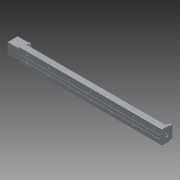
# Autodesk Inventor part: KR55A-980L-1A0-Body
Saved by Autodesk Inventor 2011 SP1 (Build 150282100, 282)
## iProperties
Created: 2013-10-23
Part Number: KR55A-980L-1A0-Body
Catalog Web Link: www.cadenas.de
Description: LM Guide Actuator - Body-KR
Vendor: THK
Document SubType Name: Modeling
Designer: PARTuser1
Manufacturer: THK
Density: 1 g/cm^3
Category: PARTsolutions
Company: THK
Title: KR55A-980L-1A0-Body
Author: Cadenas PARTsolutions
Comments: KR
PSOL_IDENT_0: {$CADENAS_DATA\23d-libs\thk\lm_guide_actuator\type_kr\parts\lm_g_a_kr_body.prj},214 {VTYP=3D},{NB=KR
PSOL_IDENT_1: 55A-980L-1A0-Body},{LINA=KR55A-980L-1A0-Body},{NN=LM Guide Actuator - Body},{DATE=10.01.2013 04:45:2
PSOL_IDENT_2: 4},{GEOMDATE=10.01.2013 04:45:00},{VERSION=},{LINEID=80},{LINESUBID=-1},{WBVAR=LM,TYPE,PC,TOHIF}  {N
PSOL_IDENT_3: B=KR55A-980L-1A0-Body},{LINA=KR55A-980L-1A0-Body},{KT=DUMMY},{ORDER=KR55},{XTYPE=8},{LM=980},{L1=108
PSOL_IDENT_4: 9},{TYPE=A},{SR=826},{H=90},{G=40},{F=200},{N=7},{N1=5},{LM1=980,1080,1180,1280,1380},{TYPE1='A','B'
PSOL_IDENT_5: },{TYPE2=2},{PC=1},{TOHIF=A0},{TOHIF1='A0','Basic Type (with Housing A, without Intermediate flange)
PSOL_IDENT_6: ','00','Old Basic Type (with Housing A, without Intermediate flange)','1[]','Administration number 1
PSOL_IDENT_7: []','0A','Administration number 0A','0B','Administration number 0B','0G','Administration number 0G'}
PSOL_IDENT_8: ,{TOB=1},{DMTR=64},{A=96},{L=976}
CNS_NT: KR
CNS_NB: KR55A-980L-1A0-Body
CNS_NBSYN: $ORDER.$TYPE.-$LM.L-$PC.$TOHIF.-Body
CNS_LINA: KR55A-980L-1A0-Body
CNS_ORDER: KR55
CNS_XTYPE: 8
CNS_LM: 980
CNS_L1: 1089.000
CNS_TYPE: A
CNS_SR: 826.000
CNS_H: 90.000
CNS_G: 40.000
CNS_F: 200.000
CNS_N: 7.000
CNS_N1: 5.000
CNS_LM1: 980,1080,1180,1280,1380
CNS_TYPE1: 'A','B'
CNS_TYPE2: 2.000
CNS_PC: Cover provided
CNS_TOHIF: Basic Type (with Housing A, without Intermediate flange)
CNS_TOHIF1: 'A0','Basic Type (with Housing A, without Intermediate flange)','00','Old Basic Type (with Housing A, without Intermediate flange)','1[]','Administration number 1[]','0A','Administration number 0A','0B','Administration number 0B','0G','Administration number 0G'
CNS_TOB: 1.000
CNS_DMTR: 64.000
CNS_A: 96.000
CNS_L: 976.000
SUPPLIER: THK
ARTICLENO: KR55A-980L-1A0-Body
BOMINFO: KR55A-980L-1A0-Body
CREATOR: CADENAS GmbH
Autodesk Inventor part; units mm, degrees
sketch "Sketch_1" plane through (0, 0, 0) normal (1, 0, 0) x (0, 1, 0)
  line L0 (-30.7, 50) -> (-32, 48.7)
  line L1 (-32, 48.7) -> (-32, 19.7)
  line L2 (-32, 19.7) -> (-31.3, 19)
  line L3 (-31.3, 19) -> (-31.3, 6.3)
  line L4 (-31.3, 6.3) -> (-32, 5.6)
  line L5 (-32, 5.6) -> (-32, -5.6)
  line L6 (-32, -5.6) -> (-31.3, -6.3)
  line L7 (-31.3, -6.3) -> (-31.3, -19)
  line L8 (-31.3, -19) -> (-32, -19.7)
  line L9 (-32, -19.7) -> (-32, -48.7)
  line L10 (-32, -48.7) -> (-30.7, -50)
  line L11 (-30.7, -50) -> (-17.5, -50)
  line L12 (-17.5, -50) -> (-17, -49.5)
  line L13 (-17, -49.5) -> (7, -49.5)
  line L14 (7, -49.5) -> (8, -48.5)
  line L15 (8, -48.5) -> (8, -36.72)
  line L16 (8, -36.72) -> (7.5, -36.22)
  line L17 (7.5, -36.22) -> (3.59, -36.22)
  line L18 (3.59, -36.22) -> (0.49, -39.32)
  line L19 (0.49, -39.32) -> (-11.32, -39.32)
  line L20 (-11.32, -39.32) -> (-14.42, -36.22)
  line L21 (-14.42, -36.22) -> (-15, -36.22)
  arc A0 (-19, -32.22) -> (-15, -36.22) centre (-15, -32.22) ccw
  line L22 (-19, -32.22) -> (-19, 32.22)
  arc A1 (-15, 36.22) -> (-19, 32.22) centre (-15, 32.22) ccw
  line L23 (-15, 36.22) -> (-14.42, 36.22)
  line L24 (-14.42, 36.22) -> (-11.32, 39.32)
  line L25 (-11.32, 39.32) -> (0.49, 39.32)
  line L26 (0.49, 39.32) -> (3.59, 36.22)
  line L27 (3.59, 36.22) -> (7.5, 36.22)
  line L28 (7.5, 36.22) -> (8, 36.72)
  line L29 (8, 36.72) -> (8, 48.5)
  line L30 (8, 48.5) -> (7, 49.5)
  line L31 (7, 49.5) -> (-17, 49.5)
  line L32 (-17, 49.5) -> (-17.5, 50)
  line L33 (-17.5, 50) -> (-30.7, 50)
  constraints: 68 end point, 4 point on circle, 2 centre point
extrude "Extrusion1" add sketch "Sketch_1" along normal blind 980
sketch "Sketch_2" plane through (0, 0, 0) normal (1, 0, 0) x (0, 1, 0)
  line L0 (23, 49.5) -> (-29.5, 49.5)
  arc A0 (-29.5, 49.5) -> (-31.5, 47.5) centre (-29.5, 47.5) ccw
  line L1 (-31.5, 47.5) -> (-31.5, -47.5)
  arc A1 (-31.5, -47.5) -> (-29.5, -49.5) centre (-29.5, -47.5) ccw
  line L2 (-29.5, -49.5) -> (23, -49.5)
  arc A2 (23, -49.5) -> (25, -47.5) centre (23, -47.5) ccw
  line L3 (25, -47.5) -> (25, -43.5)
  arc A3 (25.5, -43) -> (25, -43.5) centre (25.5, -43.5) ccw
  line L4 (25.5, -43) -> (38, -43)
  arc A4 (38, -43) -> (40, -41) centre (38, -41) ccw
  line L5 (40, -41) -> (40, 41)
  arc A5 (40, 41) -> (38, 43) centre (38, 41) ccw
  line L6 (38, 43) -> (25.5, 43)
  arc A6 (25, 43.5) -> (25.5, 43) centre (25.5, 43.5) ccw
  line L7 (25, 43.5) -> (25, 47.5)
  arc A7 (25, 47.5) -> (23, 49.5) centre (23, 47.5) ccw
  constraints: 16 end point, 16 point on circle, 8 centre point
extrude "Extrusion2" add sketch "Sketch_2" against normal blind 15
sketch "Sketch_17" plane through (0, 0, 0) normal (1, 0, 0) x (0, 1, 0)
  line L0 (37, 39) -> (-29.5, 39)
  arc A0 (-29.5, 39) -> (-31.5, 37) centre (-29.5, 37) ccw
  line L1 (-31.5, 37) -> (-31.5, -37)
  arc A1 (-31.5, -37) -> (-29.5, -39) centre (-29.5, -37) ccw
  line L2 (-29.5, -39) -> (37, -39)
  arc A2 (37, -39) -> (40, -36) centre (37, -36) ccw
  line L3 (40, -36) -> (40, 36)
  arc A3 (40, 36) -> (37, 39) centre (37, 36) ccw
  constraints: 8 end point, 8 point on circle, 4 centre point
extrude "Extrusion3" add sketch "Sketch_17" against normal blind 94
sketch "Sketch_3" plane through (0, 0, 0) normal (1, 0, 0) x (0, 1, 0)
  arc A0 (18, 24) -> (-18, 24) centre (0, 0) ccw
  line L0 (-18, 24) -> (-18, -24)
  arc A1 (-18, -24) -> (18, -24) centre (0, 0) ccw
  line L1 (18, -24) -> (18, 24)
  constraints: 4 end point, 4 point on circle, 2 centre point
extrude "Extrusion4" add sketch "Sketch_3" along normal blind 5
sketch "Sketch_4" plane through (0, 0, 0) normal (1, 0, 0) x (0, 1, 0)
  arc A0 (8, 25.7876) -> (-8, 25.7876) centre (0, 0) ccw
  line L0 (-8, 25.7876) -> (-8, 14.8866)
  arc A1 (8, 14.8866) -> (-8, 14.8866) centre (0, 0) ccw
  line L1 (8, 14.8866) -> (8, 25.7876)
  constraints: 4 end point, 4 point on circle, 2 centre point
extrude "Extrusion5" add sketch "Sketch_4" along normal blind 15
sketch "Sketch_26" plane through (0, 0, 0) normal (1, 0, 0) x (0, 1, 0)
  arc A0 (-8, -14.8866) -> (8, -14.8866) centre (0, 0) ccw
  line L0 (-8, -14.8866) -> (-8, -25.7876)
  arc A1 (-8, -25.7876) -> (8, -25.7876) centre (0, 0) ccw
  line L1 (8, -25.7876) -> (8, -14.8866)
  constraints: 4 end point, 4 point on circle, 2 centre point
extrude "Extrusion6" add sketch "Sketch_26" along normal blind 15
sketch "Sketch_38" plane through (0, 12.5, 0) normal (0, 1, 0) x (1, 0, 0)
  line L0 (10, -21.65) -> (5, -21.65)
  line L1 (5, -21.65) -> (5, -17.4)
  line L2 (5, -17.4) -> (9.8, -17.4)
  arc A0 (10, -17.6) -> (9.8, -17.4) centre (9.8, -17.6) ccw
  line L3 (10, -17.6) -> (10, -21.65)
  line L4 (10, -21.65) -> (5, -21.65)
  constraints: 10 end point, 2 point on circle, 1 centre point
revolve "Revolution1" add sketch "Sketch_38" angle 360 about axis through (10, 12.5, 21.65) along (1, 0, 0)
pattern_linear "Rectangular Pattern1" count 2 spacing 43.3 along (0, 0, -1) count 2 spacing 25 along (0, -1, 0) of "Revolution1"
sketch "Sketch_7" plane through (980, 0, 0) normal (1, 0, 0) x (0, 0, -1)
  line L0 (-50, 38.35) -> (-50, -29.85)
  arc A0 (-50, -29.85) -> (-48.35, -31.5) centre (-48.35, -29.85) ccw
  line L1 (-48.35, -31.5) -> (48.35, -31.5)
  arc A1 (48.35, -31.5) -> (50, -29.85) centre (48.35, -29.85) ccw
  line L2 (50, -29.85) -> (50, 38.35)
  arc A2 (50, 38.35) -> (48.35, 40) centre (48.35, 38.35) ccw
  line L3 (48.35, 40) -> (-48.35, 40)
  arc A3 (-48.35, 40) -> (-50, 38.35) centre (-48.35, 38.35) ccw
  constraints: 8 end point, 8 point on circle, 4 centre point
extrude "Extrusion7" add sketch "Sketch_7" along normal blind 15
sketch "Sketch_20" plane through (980, 0, 0) normal (1, 0, 0) x (0, 0, -1)
  line L0 (-55, 18) -> (-43, 18)
  line L1 (-43, 18) -> (-43, 38.35)
  arc A0 (-41.35, 40) -> (-43, 38.35) centre (-41.35, 38.35) ccw
  line L2 (-41.35, 40) -> (41.35, 40)
  arc A1 (43, 38.35) -> (41.35, 40) centre (41.35, 38.35) ccw
  line L3 (43, 38.35) -> (43, 18)
  line L4 (43, 18) -> (55, 18)
  line L5 (55, 18) -> (55, 48)
  line L6 (55, 48) -> (-55, 48)
  line L7 (-55, 48) -> (-55, 18)
  constraints: 16 end point, 4 point on circle, 2 centre point
extrude "Extrusion8" cut sketch "Sketch_20" along normal blind 20
sketch "Sketch_23" plane through (0, 0, 0) normal (0, 0, 1) x (1, 0, 0)
  line L0 (984, 0) -> (979, 0)
  line L1 (979, 0) -> (979, 15)
  line L2 (979, 15) -> (984, 15)
  line L3 (984, 15) -> (984, 0)
  line L4 (984, 0) -> (979, 0)
  constraints: 10 end point
revolve "Revolution2" cut sketch "Sketch_23" angle 360 about axis through (984, 0, 0) along (1, 0, 0)
sketch "Sketch_8" plane through (0, -5, 0) normal (0, 1, 0) x (1, 0, 0)
  line L0 (980, 25) -> (969, 25)
  line L1 (969, 25) -> (969, 32)
  line L2 (969, 32) -> (980, 34)
  line L3 (980, 34) -> (980, 25)
  line L4 (980, 25) -> (969, 25)
  constraints: 10 end point
revolve "Revolution3" add sketch "Sketch_8" angle 360 about axis through (980, -5, -25) along (1, 0, 0)
sketch "Sketch_41" plane through (0, -5, 0) normal (0, 1, 0) x (1, 0, 0)
  line L0 (980, -25) -> (969, -25)
  line L1 (969, -25) -> (969, -18)
  line L2 (969, -18) -> (980, -16)
  line L3 (980, -16) -> (980, -25)
  line L4 (980, -25) -> (969, -25)
  constraints: 10 end point
revolve "Revolution4" add sketch "Sketch_41" angle 360 about axis through (980, -5, 25) along (1, 0, 0)
sketch "Sketch_9" plane through (0, 0, 0) normal (0, 0, 1) x (1, 0, 0)
  line L0 (984, 0) -> (4, 0)
  line L1 (4, 0) -> (4, 10)
  line L2 (4, 10) -> (984, 10)
  line L3 (984, 10) -> (984, 0)
  line L4 (984, 0) -> (4, 0)
  constraints: 10 end point
revolve "Revolution5" add sketch "Sketch_9" angle 360 about axis through (984, 0, 0) along (1, 0, 0)
sketch "Sketch14" plane through (995, 0, 0) normal (1, 0, 0) x (0, 0, -1)
  point P0 (-44.5, -26)
hole "Drilling 2" at (995, -26, 44.5) direction (-1, 0, 0) diameter 7.7 depth 3
pattern_linear "Rectangular Pattern2" count 2 spacing 89 along (0, 0, -1) count 3 spacing 15 along (0, 1, 0) of "Drilling 2"
sketch "Sketch_11" plane through (0, -26, 0) normal (0, 1, 0) x (1, 0, 0)
  line L0 (995, -44.5) -> (991.3, -44.5)
  line L1 (991.3, -44.5) -> (991.3, -41)
  line L2 (991.3, -41) -> (994.8, -41)
  arc A0 (995, -41.2) -> (994.8, -41) centre (994.8, -41.2) ccw
  line L3 (995, -41.2) -> (995, -44.5)
  line L4 (995, -44.5) -> (991.3, -44.5)
  constraints: 10 end point, 2 point on circle, 1 centre point
revolve "Revolution6" add sketch "Sketch_11" angle 360 about axis through (995, -26, 44.5) along (1, 0, 0)
pattern_linear "Rectangular Pattern3" count 2 spacing 89 along (0, 0, -1) count 3 spacing 15 along (0, 1, 0) of "Revolution6"
sketch "Sketch_13" plane through (0, -27, 0) normal (0, 1, 0) x (1, 0, 0)
  arc A0 (-72, -19) -> (-62, -29) centre (-62, -19) ccw
  line L0 (-62, -29) -> (-37, -29)
  arc A1 (-37, -29) -> (-27, -19) centre (-37, -19) ccw
  line L1 (-27, -19) -> (-27, 19)
  arc A2 (-27, 19) -> (-37, 29) centre (-37, 19) ccw
  line L2 (-37, 29) -> (-62, 29)
  arc A3 (-62, 29) -> (-72, 19) centre (-62, 19) ccw
  line L3 (-72, 19) -> (-72, -19)
  constraints: 8 end point, 8 point on circle, 4 centre point
extrude "Extrusion9" cut sketch "Sketch_13" along normal blind 72
sketch "Sketch_39" plane through (0, 0, 0) normal (0, 1, 0) x (-1, 0, 0)
  line L0 (-996, 0) -> (-991, 0)
  line L1 (-994, 0) -> (-994, -7.5)
  line L2 (-994, -7.5) -> (-993, -8.5)
  line L3 (-993, -8.5) -> (-991, -8.5)
  line L4 (-991, -8.5) -> (-991, -15)
  line L5 (-991, -15) -> (-996, -15)
  line L6 (-996, -15) -> (-996, 0)
  line L7 (-996, 0) -> (-994, 0)
  constraints: 16 end point
revolve "Revolution7" cut sketch "Sketch_39" angle 360 about axis through (996, 0, 0) along (1, 0, 0)
sketch "Sketch_18" plane through (0, 0, 0) normal (0, 0, 1) x (1, 0, 0)
  line L0 (-65, 0) -> (-95, 0)
  line L1 (-95, 0) -> (-95, 25)
  line L2 (-95, 25) -> (-65, 25)
  line L3 (-65, 25) -> (-65, 0)
  line L4 (-65, 0) -> (-95, 0)
  constraints: 10 end point
revolve "Revolution8" cut sketch "Sketch_18" angle 360 about axis through (-65, 0, 0) along (1, 0, 0)
sketch "Sketch_19" plane through (0, -26, 0) normal (0, 1, 0) x (1, 0, 0)
  line L0 (-15, -44.5) -> (-20, -44.5)
  line L1 (-20, -44.5) -> (-20, -40.45)
  arc A0 (-19.8, -40.25) -> (-20, -40.45) centre (-19.8, -40.45) ccw
  line L2 (-19.8, -40.25) -> (-15, -40.25)
  line L3 (-15, -40.25) -> (-15, -44.5)
  line L4 (-15, -44.5) -> (-20, -44.5)
  constraints: 10 end point, 2 point on circle, 1 centre point
revolve "Revolution9" add sketch "Sketch_19" angle 360 about axis through (-15, -26, 44.5) along (1, 0, 0)
pattern_linear "Rectangular Pattern4" count 2 spacing 89 along (0, 0, -1) count 3 spacing 15 along (0, 1, 0) of "Revolution9"
sketch "Sketch_21" plane through (0, 0, 0) normal (0, 0, 1) x (1, 0, 0)
  line L0 (-27, 0) -> (-59, 0)
  line L1 (-59, 0) -> (-59, 5)
  line L2 (-59, 5) -> (-58, 6)
  line L3 (-58, 6) -> (-37, 6)
  line L4 (-37, 6) -> (-37, 6.5)
  line L5 (-37, 6.5) -> (-36, 7.5)
  line L6 (-36, 7.5) -> (-35, 7.5)
  line L7 (-35, 7.5) -> (-35, 11.5)
  line L8 (-35, 11.5) -> (-34, 12.5)
  line L9 (-34, 12.5) -> (-29, 12.5)
  line L10 (-29, 12.5) -> (-28, 11.5)
  line L11 (-28, 11.5) -> (-28, 10)
  line L12 (-28, 10) -> (-27, 10)
  line L13 (-27, 10) -> (-27, 0)
  line L14 (-27, 0) -> (-59, 0)
  constraints: 30 end point
revolve "Revolution10" add sketch "Sketch_21" angle 360 about axis through (-27, 0, 0) along (1, 0, 0)
sketch "Sketch_22" plane through (-27, 0, 0) normal (1, 0, 0) x (0, 0, -1)
  circle A0 centre (0, 0) radius 16
  line L0 (-15.5563, 0) -> (0, -15.5563)
  line L1 (0, -15.5563) -> (15.5563, 0)
  line L2 (15.5563, 0) -> (0, 15.5563)
  line L3 (0, 15.5563) -> (-15.5563, 0)
  constraints: 8 end point, 1 centre point
extrude "Extrusion10" cut sketch "Sketch_22" against normal blind 15
sketch "Sketch_37" plane through (0, 0, 0) normal (0, 0, 1) x (1, 0, 0)
  line L0 (-31.5, 11.5) -> (-31.5, 13)
  line L1 (-31.5, 13) -> (-29, 13)
  line L2 (-29, 13) -> (-29, 11.5)
  line L3 (-29, 11.5) -> (-31.5, 11.5)
  line L4 (-31.5, 11.5) -> (-31.5, 13)
  constraints: 10 end point
revolve "Revolution11" cut sketch "Sketch_37" angle 360 about axis through (-31.5, 11.5, 0) along (0, -1, 0)
sketch "Sketch23" plane through (-94, 0, 0) normal (-1, 0, 0) x (0, 0, 1)
  point P0 (-24.7487, 24.7487)
hole "Drilling 5" at (-94, 24.7487, -24.7487) direction (1, 0, 0) diameter 4.134 depth 12 tip angle 140 countersink diameter 5 countersink angle 90 thread size "M5x0.8" class "6H" standard "ISO Metric profile"
pattern_linear "Rectangular Pattern5" count 2 spacing 49.4975 along (0, 0, 1) count 2 spacing 49.4975 along (0, -1, 0) of "Drilling 5"
sketch "Sketch24" plane through (-15, -29.5, -49.5) normal (0, 0, -1) x (-1, 0, 0)
  point P0 (-105, 24.5)
hole "Drilling 6" at (90, -5, -49.5) direction (0, 0, 1) diameter 2.1129 depth 5 tip angle 140 countersink diameter 2.6 countersink angle 90 thread size "M2.6x0.45" class "6H" standard "ISO Metric profile"
pattern_linear "Rectangular Pattern6" count 5 spacing 200 along (1, 0, 0) of "Drilling 6"
sketch "Sketch25" plane through (-15, -29.5, 49.5) normal (0, 0, 1) x (1, 0, 0)
  point P0 (105, 24.5)
hole "Drilling 7" at (90, -5, 49.5) direction (0, 0, -1) diameter 2.1129 depth 5 tip angle 140 countersink diameter 2.6 countersink angle 90 thread size "M2.6x0.45" class "6H" standard "ISO Metric profile"
pattern_linear "Rectangular Pattern7" count 5 spacing 200 along (1, 0, 0) of "Drilling 7"
sketch "Sketch26" plane through (-15, 40, 41) normal (0, 1, 0) x (1, 0, 0)
  point P0 (7.42, 66)
hole "Drilling 8" at (-7.58, 40, -25) direction (0, -1, 0) diameter 2.1129 depth 5 tip angle 140 countersink diameter 2.6 countersink angle 90 thread size "M2.6x0.45" class "6H" standard "ISO Metric profile"
sketch "Sketch27" plane through (-15, 40, 41) normal (0, 1, 0) x (1, 0, 0)
  point P0 (7.42, 16)
hole "Drilling 9" at (-7.58, 40, 25) direction (0, -1, 0) diameter 2.1129 depth 5 tip angle 140 countersink diameter 2.6 countersink angle 90 thread size "M2.6x0.45" class "6H" standard "ISO Metric profile"
sketch "Sketch_29" plane through (40, 0, 0) normal (1, 0, 0) x (0, 0, -1)
  line L0 (-25, -18) -> (-25, -33)
  line L1 (-25, -33) -> (-29.5, -33)
  line L2 (-29.5, -33) -> (-29.5, -27.6)
  line L3 (-29.5, -27.6) -> (-32, -27.6)
  line L4 (-32, -27.6) -> (-32, -18)
  line L5 (-32, -18) -> (-25, -18)
  line L6 (-25, -18) -> (-25, -33)
  constraints: 14 end point
revolve "Revolution12" cut sketch "Sketch_29" angle 360 about axis through (40, -18, 25) along (0, 1, 0)
pattern_linear "Rectangular Pattern8" count 7 spacing 150 along (1, 0, 0) of "Revolution12"
sketch "Sketch_31" plane through (40, 0, 0) normal (1, 0, 0) x (0, 0, -1)
  line L0 (25, -18) -> (25, -33)
  line L1 (25, -33) -> (20.5, -33)
  line L2 (20.5, -33) -> (20.5, -27.6)
  line L3 (20.5, -27.6) -> (18, -27.6)
  line L4 (18, -27.6) -> (18, -18)
  line L5 (18, -18) -> (25, -18)
  line L6 (25, -18) -> (25, -33)
  constraints: 14 end point
revolve "Revolution13" cut sketch "Sketch_31" angle 360 about axis through (40, -18, -25) along (0, 1, 0)
pattern_linear "Rectangular Pattern9" count 7 spacing 150 along (1, 0, 0) of "Revolution13"
ref_plane "body_dummy_XY" through (0, 0, 0) normal (1, 0, 0) x (0, 0, -1)
ref_plane "body_dummy_YZ" through (0, 0, 0) normal (0, 0, -1) x (0, 1, 0)
ref_plane "body_dummy_ZX" through (0, 0, 0) normal (0, 1, 0) x (1, 0, 0)
ref_plane "body_flange_XY" through (-94, 0, 0) normal (1, 0, 0) x (0, 0, -1)
ref_plane "body_flange_YZ" through (-94, 0, 0) normal (0, 0, -1) x (0, 1, 0)
ref_plane "body_flange_ZX" through (-94, 0, 0) normal (0, 1, 0) x (1, 0, 0)
ref_plane "body_pc_XY" through (-7.58, 40, 0) normal (1, 0, 0) x (0, 0, -1)
ref_plane "body_pc_YZ" through (-7.58, 40, 0) normal (0, 0, -1) x (0, 1, 0)
ref_plane "body_pc_ZX" through (-7.58, 40, 0) normal (0, 1, 0) x (1, 0, 0)
ref_plane "body_sensor_rail_XY" through (490, -5, 49.5) normal (0, 0, 1) x (1, 0, 0)
ref_plane "body_sensor_rail_YZ" through (490, -5, 49.5) normal (1, 0, 0) x (0, 1, 0)
ref_plane "body_sensor_rail_ZX" through (490, -5, 49.5) normal (0, 1, 0) x (0, 0, 1)
ref_plane "body_sensor_rail2_XY" through (490, -5, -49.5) normal (0, 0, 1) x (1, 0, 0)
ref_plane "body_sensor_rail2_YZ" through (490, -5, -49.5) normal (1, 0, 0) x (0, 1, 0)
ref_plane "body_sensor_rail2_ZX" through (490, -5, -49.5) normal (0, 1, 0) x (0, 0, 1)
ref_plane "body_slider_XY" through (15, 0, 0) normal (1, 0, 0) x (0, 0, -1)
ref_plane "body_slider_YZ" through (15, 0, 0) normal (0, 0, -1) x (0, 1, 0)
ref_plane "body_slider_ZX" through (15, 0, 0) normal (0, 1, 0) x (1, 0, 0)
ref_plane "body_slider2_XY" through (969, 0, 0) normal (1, 0, 0) x (0, 0, -1)
ref_plane "body_slider2_YZ" through (969, 0, 0) normal (0, 0, -1) x (0, 1, 0)
ref_plane "body_slider2_ZX" through (969, 0, 0) normal (0, 1, 0) x (1, 0, 0)
body "Solid1"
